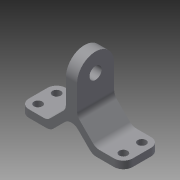
# Autodesk Inventor part: clip_base
Saved by Autodesk Inventor 2013 (Build 170138000, 138)
## iProperties
Created: 2013-03-18
Part Number: clip_base
Material: Generic
Document SubType Name: Modeling
Designer: Mahisorn
Density: 1 g/cm^3
Author: Mahisorn
Autodesk Inventor part; units mm, degrees
ref_plane "YZ Plane" through (0, 0, 0) normal (1, 0, 0) x (0, 1, 0)
ref_plane "XZ Plane" through (0, 0, 0) normal (0, 1, 0) x (-1, 0, 0)
ref_plane "XY Plane" through (0, 0, 0) normal (0, 0, 1) x (1, 0, 0)
sketch "Sketch1" plane through (0, 0, 0) normal (0, 1, 0) x (-1, 0, 0)
  line L0 (0, 25) -> (-3, 25)
  line L1 (-3, 25) -> (-3, 0)
  line L2 (-3, 0) -> (-13, -10)
  line L3 (-13, -10) -> (-28, -10)
  line L4 (-28, -14) -> (-11.3431, -14)
  line L5 (-11.3431, -14) -> (0, -2.6569)
  line L6 (0, 25) -> (0, -2.6569)
  line L7 (-28, -10) -> (-28, -14)
  dimension "d4" = 3
  dimension "d6" = 135
  dimension "d7" = 15
  dimension "d9" = 4
  dimension "d10" = 25
  dimension "d38" = 10
  dimension "d39" = 4
  constraints: 16 end point, 3 parallel, 2 perpendicular, 2 vertical
  measures "d4" distance of L0.start L0.end
  measures "d6" angle of L1 L2
  measures "d7" distance of L2.end L3.end
  measures "d9" distance between parallel lines of L5 L2
  measures "d10" distance from line of L1.end L0
  measures "d38" horizontal distance of L2.end L1.end
  measures "d39" distance of L3.end L4.start
extrude "Extrusion1" add sketch "Sketch1" along normal blind 20
fillet "Fillet1" radius 10 2 edges at (1.5, 20, 25) (1.5, 0, 25)
sketch "Sketch3" plane through (3, 0, 0) normal (1, 0, 0) x (0, 0, -1)
  arc A0 (-15, 20) -> (-15, 0) centre (-15, 10) ccw projected
  constraints: 1 coincident
hole "Hole2" at (3, 10, 15) direction (-1, 0, 0) diameter 6.6 end through all clearance for "Flat Head Machine Screw" size "M6" standard "Ansi Metric M Profile"
sketch "Sketch4" plane through (13, 0, -10) normal (0, 0, 1) x (1, 0, 0)
  line L0 (0, 20) -> (15, 20) projected
  line L1 (15, 0) -> (15, 20) projected
  point P0 (-13, 0)
  point P1 (10, 15)
  point P2 (10, 5)
  dimension "d28" = 5
  dimension "d29" = 10
  dimension "d40" = 5
  constraints: 1 vertical alignment
  measures "d28" distance from line of point (10, 15) L0
  measures "d29" distance of point (10, 5) point (10, 15)
  measures "d40" distance from line of L1 point (10, 15)
hole "Hole3" at (23, 15, -10) at (23, 5, -10) direction (0, 0, -1) diameter 4.5 end through all clearance for "Flat Head Machine Screw" size "M4" standard "Ansi Metric M Profile"
fillet "Fillet4" radius 5 5 edges at (28, 20, -12) (28, 0, -12) (13, 10, -10) (11.3431, 10, -14) (3, 10, 0)
mirror "Mirror2" about plane through (0, 0, -2.6569) normal (-1, 0, 0) of "Fillet4", "Extrusion1", "Hole3", "Hole2", "Fillet1"
fillet "Fillet5" radius 5 1 edges at (0, 10, -2.6569)
body "Solid1"
